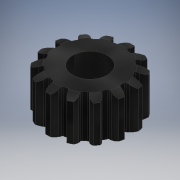
# Autodesk Inventor part: Engrenage bol
Saved by Autodesk Inventor 2017 (Build 210142000, 142)
## iProperties
Company: FABLAB FrenchMakers
Part Number: Engrenage bol
Material: Acier inoxydable
Document SubType Name: Modeling
Designer: FABLAB FrenchMakers
Density: 8 g/cm^3
Appearance: Asphalte 2
Mass: 14.643 g
Surface Area: 15.8008 cm^2
Volume: 1.83037 cm^3
Stock Number: 1400-01-21
Author: Adrien MARY
Autodesk Inventor part; units mm, degrees
ref_plane "YZ Plane" through (0, 0, 0) normal (1, 0, 0) x (0, 1, 0)
ref_plane "XZ Plane" through (0, 0, 0) normal (0, 1, 0) x (-1, 0, 0)
ref_plane "XY Plane" through (0, 0, 0) normal (0, 0, 1) x (1, 0, 0)
sketch "Esquisse1" plane through (0, 0, 0) normal (0, 0, 1) x (1, 0, 0)
  circle A0 centre (0, 0) radius 7.5
  dimension "d0" = 15
  constraints: 1 centre point, 1 coincident
  measures "d0" diameter of A0
extrude "Extrusion1" add sketch "Esquisse1" along normal mid plane 10
sketch "Esquisse3" plane through (0, 0, 5) normal (0, 0, 1) x (1, 0, 0)
  line L0 (-1, 7.6485) -> (-1, 8.4018)
  arc A0 (-0.4805, 9.9585) -> (-1, 8.4018) centre (1.7495, 8.3493) ccw
  line L1 (-0.3994, 10) -> (0, 10)
  line L2 (0, 0) -> (0, 12.4164)
  arc A1 (-0.3994, 10) -> (-0.4805, 9.9585) centre (-0.3994, 9.9) ccw
  arc A2 (-1.2097, 7.4018) -> (-1, 7.6485) centre (-1.25, 7.6485) ccw
  circle A3 centre (0, 0) radius 7.5 construction
  line L3 (1, 7.6485) -> (1, 8.4018)
  arc A4 (1, 8.4018) -> (0.4805, 9.9585) centre (-1.7495, 8.3493) ccw
  arc A5 (0.4805, 9.9585) -> (0.3994, 10) centre (0.3994, 9.9) ccw
  arc A6 (1, 7.6485) -> (1.2097, 7.4018) centre (1.25, 7.6485) ccw
  arc A7 (1.2097, 7.4018) -> (-1.2097, 7.4018) centre (0, 0) ccw
  line L4 (0, 10) -> (0.3994, 10)
  point P0 (-1, 7.8392)
  point P1 (-0.45, 10)
  point P2 (1, 7.8392)
  point P3 (0.45, 10)
  dimension "d9" = 10
  dimension "d10" = 2
  dimension "d12" = 0.9
  dimension "d13" = 2.75
  dimension "d14" = 0.1
  dimension "d16" = 0.25
  dimension "d17" = 1
  constraints: 16 point on circle, 10 end point, 10 symmetric about line, 7 centre point, 4 point on line, 3 tangent, 1 coincident, 1 horizontal, 1 vertical, 6 other
  measures "d9" distance from line of point (0, 0) L1
  measures "d10" diameter of L0 L2
  measures "d12" diameter of point (-0.45, 10) L2
  measures "d13" radius of A0
  measures "d14" radius of A1
  measures "d16" radius of A2
  measures "d17" vertical distance of A2.start L0.end
extrude "Extrusion2" add sketch "Esquisse3" against normal up to surface (10 mm away)
pattern_circular "Réseau circulaire1" count 14 over 360 about axis through (0, 0, 0) along (0, 0, 1) of "Extrusion2"
sketch "Esquisse12" plane through (0, 0, 5) normal (0, 0, 1) x (1, 0, 0)
  point P0 (0, 0)
  point P1 (0, 0)
  constraints: 1 coincident
hole "Perçage5" at (0, 0, 5) direction (0, 0, -1) diameter 8 end through all
sketch "Esquisse13" plane through (0, 0, 0) normal (0, 1, 0) x (-1, 0, 0)
  line L0 (-5.9453, 5) -> (-5.3564, 5) projected
  line L1 (-7.8158, 5) -> (-9.8158, 4.2721)
  line L2 (-9.8158, 4.2721) -> (-9.8158, -4.2721)
  line L3 (-9.8158, -4.2721) -> (-7.8158, -5)
  line L4 (-5.3564, -5) -> (-5.9453, -5) projected
  line L5 (-11.8158, -5) -> (-7.8158, -5)
  line L6 (-11.8158, -5) -> (-11.8158, 5)
  line L7 (-11.8158, 5) -> (-7.8158, 5)
  line L8 (-6.6034, 5) -> (-7.1923, 5) projected
  line L9 (-9.8158, 5) -> (-9.8158, -5) projected
  line L10 (-7.1923, -5) -> (-6.6034, -5) projected
  line L11 (0, -7) -> (0, 7) projected
  point P0 (0, 0)
  dimension "d96" = 2
  dimension "d97" = 20
  dimension "d98" = 20
  dimension "d99" = 2
  constraints: 12 end point, 3 collinear, 2 vertical, 1 point on line, 1 vertical alignment
  measures "d96" distance between parallel lines of L2 L6
  measures "d97" angle of L7 L1
  measures "d98" angle of L5 L3
  measures "d99" distance from line of L2 L1.start
revolve "Révolution2" cut sketch "Esquisse13" angle 360 about axis through (0, 0, -10) along (0, 0, 1)
equation "\"d98\" = d97"
equation "\"nombredor\" = 1.61803"
equation "\"pi\" = 3.141593"
